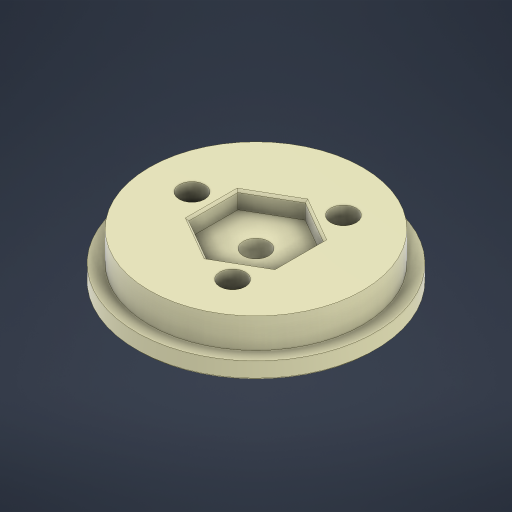
# Autodesk Inventor part: Shaft2_Joint2
Saved by Autodesk Inventor 2023 (Build 270158000, 158)
## iProperties
Created: 2023-02-21
Part Number: Shaft2_Joint2
Material: ABS Plastic
Document SubType Name: Modeling
Designer: dzw04
Density: 1.06 g/cm^3
Appearance: Smooth - Ash
Author: dzw04
Autodesk Inventor part; units mm, degrees
ref_plane "YZ Plane" through (0, 0, 0) normal (1, 0, 0) x (0, 1, 0)
ref_plane "XZ Plane" through (0, 0, 0) normal (0, 1, 0) x (-1, 0, 0)
ref_plane "XY Plane" through (0, 0, 0) normal (0, 0, 1) x (1, 0, 0)
sketch "Sketch1" plane through (0, 0, 0) normal (0, 1, 0) x (-1, 0, 0)
  circle A0 centre (0, 0) radius 14
  dimension "d0" = 28
  constraints: 1 centre point, 1 coincident
  measures "d0" diameter of A0
extrude "Extrusion1" add sketch "Sketch1" along normal blind 2
sketch "Sketch2" plane through (0, 2, 0) normal (0, 1, 0) x (1, 0, 0)
  circle A0 centre (0, 0) radius 12.5
  dimension "d3" = 25
  constraints: 1 centre point, 1 coincident
  measures "d3" diameter of A0
extrude "Extrusion2" add sketch "Sketch2" along normal blind 3.5
sketch "Sketch3" plane through (0, 5.5, 0) normal (0, 1, 0) x (1, 0, 0)
  line L0 (5, -2.8868) -> (0, -5.7735)
  line L1 (0, -5.7735) -> (-5, -2.8868)
  line L2 (-5, -2.8868) -> (-5, 2.8868)
  line L3 (-5, 2.8868) -> (0, 5.7735)
  line L4 (0, 5.7735) -> (5, 2.8868)
  line L5 (5, 2.8868) -> (5, -2.8868)
  point P0 (0, 0)
  point P1 (0, 0)
  dimension "d6" = 10
  constraints: 12 end point, 1 coincident, 1 vertical, 13 other
  measures "d6" distance between parallel lines of L3 L0
extrude "Extrusion3" cut sketch "Sketch3" against normal blind 2
sketch "Sketch4" plane through (0, 5.5, 0) normal (0, 1, 0) x (1, 0, 0)
  circle A0 centre (0, 0) radius 1.5
  circle A1 centre (0, 0) radius 7.5 construction
  circle A2 centre (-7.5, 0) radius 1.5
  circle A3 centre (-3.75, -6.4952) radius 1.5
  circle A4 centre (3.75, -6.4952) radius 1.5
  circle A5 centre (7.5, 0) radius 1.5
  circle A6 centre (3.75, 6.4952) radius 1.5
  circle A7 centre (-3.75, 6.4952) radius 1.5
  dimension "d13" = 15
  dimension "d12" = 3
  dimension "d14" = 3
  dimension "d17" = 360
  constraints: 7 centre point, 2 coincident, 1 horizontal alignment, 15 other
  measures "d12" diameter of A0
  measures "d14" diameter of A2
extrude "Extrusion4" cut sketch "Sketch4" against normal through all contours A0 | A2 | A4 | A6
chamfer "Chamfer2" distance 0.25 angle 45 1 edges at (14, 0, 0)
chamfer "Chamfer3" distance 0.25 angle 45 6 edges at (-5, 5.5, 0) (-2.5, 5.5, 4.3301) (2.5, 5.5, 4.3301) (5, 5.5, 0) (2.5, 5.5, -4.3301) (-2.5, 5.5, -4.3301)
body "Solid1"
